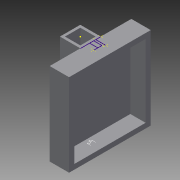
# Autodesk Inventor part: CouterWeightLink
Saved by Autodesk Inventor 2015 (Build 190159000, 159)
## iProperties
Created: 2016-03-24
Part Number: CouterWeightLink
Material: Generic
Document SubType Name: Modeling
Designer: Hatch
Density: 1 g/cm^3
Appearance: Default
Author: Hatch
Autodesk Inventor part; units mm, degrees
ref_plane "YZ Plane" through (0, 0, 0) normal (1, 0, 0) x (0, 1, 0)
ref_plane "XZ Plane" through (0, 0, 0) normal (0, 1, 0) x (-1, 0, 0)
ref_plane "XY Plane" through (0, 0, 0) normal (0, 0, 1) x (1, 0, 0)
sketch "Sketch1" plane through (0, 0, 0) normal (0, 1, 0) x (-1, 0, 0)
  line L0 (-7.25, 7.25) -> (7.25, 7.25)
  line L1 (7.25, 7.25) -> (7.25, -7.25)
  line L2 (7.25, -7.25) -> (-7.25, -7.25)
  line L3 (-7.25, -7.25) -> (-7.25, 7.25)
  line L4 (-7.25, 7.25) -> (7.25, -7.25) construction
  line L5 (7.25, 7.25) -> (-7.25, -7.25) construction
  point P0 (0, 0)
  dimension "d0" = 14.5
  dimension "d1" = 14.5
  constraints: 12 end point, 2 midpoint, 2 parallel, 1 horizontal, 1 perpendicular
  measures "d0" distance of L1.end L2.end
  measures "d1" distance of L0.end L1.end
extrude "Extrusion1" add sketch "Sketch1" along normal blind 76.2
sketch "Sketch2" plane through (0, 76.2, 0) normal (0, 1, 0) x (1, 0, 0)
  line L0 (10, -10) -> (-10, -10)
  line L1 (-10, -10) -> (-10, 10)
  line L2 (-10, 10) -> (10, 10)
  line L3 (10, 10) -> (10, -10)
  line L4 (10, -10) -> (-10, 10) construction
  line L5 (-10, -10) -> (10, 10) construction
  point P0 (0, 0)
  dimension "d4" = 20
  dimension "d5" = 20
  constraints: 12 end point, 2 midpoint, 2 parallel, 1 horizontal, 1 perpendicular
  measures "d4" distance of L1.end L2.end
  measures "d5" distance of L0.end L1.end
extrude "Extrusion2" add sketch "Sketch2" along normal blind 5
sketch "Sketch3" plane through (0, 81.2, 0) normal (0, 1, 0) x (1, 0, 0)
  line L0 (7.5, -7.5) -> (-7.5, -7.5)
  line L1 (-7.5, -7.5) -> (-7.5, 7.5)
  line L2 (-7.5, 7.5) -> (7.5, 7.5)
  line L3 (7.5, 7.5) -> (7.5, -7.5)
  line L4 (7.5, -7.5) -> (-7.5, 7.5) construction
  line L5 (-7.5, -7.5) -> (7.5, 7.5) construction
  line L6 (10, -10) -> (-10, -10)
  line L7 (-10, -10) -> (-10, 10)
  line L8 (-10, 10) -> (10, 10)
  line L9 (10, 10) -> (10, -10)
  line L10 (10, -10) -> (-10, 10) construction
  line L11 (-10, -10) -> (10, 10) construction
  point P0 (0, 0)
  dimension "d8" = 15
  dimension "d9" = 15
  constraints: 24 end point, 4 midpoint, 4 parallel, 2 horizontal, 2 perpendicular
  measures "d8" distance of L1.end L2.end
  measures "d9" distance of L0.end L1.end
extrude "Extrusion3" add sketch "Sketch3" along normal blind 76.2
sketch "Sketch4" plane through (10, 76.2, 10) normal (1, 0, 0) x (0, 0, -1)
  line L0 (20, 0) -> (20, 81.2) projected
  line L1 (15, 81.2) -> (15, 0)
  line L2 (0, 0) -> (20, 0) projected
  line L3 (15, 81.2) -> (13, 81.2)
  line L4 (17.5, 81.2) -> (2.5, 81.2) projected
  line L5 (13, 81.2) -> (13, 0)
  line L6 (13, 0) -> (15, 0)
  line L7 (20, 81.2) -> (0, 81.2) projected
  point P0 (10, -76.2)
  dimension "d12" = 2
  constraints: 8 end point, 3 point on line, 1 parallel, 1 perpendicular, 1 vertical
  measures "d12" distance of L1.start L3.end
extrude "Extrusion4" add sketch "Sketch4" along normal blind 10 contours L2 L5 L3 L1
sketch "Sketch5" plane through (10, 76.2, -3) normal (0, 0, 1) x (1, 0, 0)
  line L0 (0, 81.2) -> (10, 81.2) projected
  line L1 (10, 81.2) -> (8, 81.2)
  line L2 (8, 81.2) -> (8, 0)
  line L3 (8, 0) -> (10, 0)
  line L4 (10, 0) -> (10, 81.2)
  point P0 (-10, -76.2)
  dimension "d15" = 2
  constraints: 8 end point, 2 parallel, 1 perpendicular, 1 point on line
  measures "d15" distance of L0.end L1.end
extrude "Extrusion5" add sketch "Sketch5" along normal blind 8
sketch "Sketch6" plane through (20, 76.2, 10) normal (1, 0, 0) x (0, 0, -1)
  line L0 (5, 81.2) -> (3, 81.2)
  line L1 (3, 81.2) -> (3, 0)
  line L2 (3, 0) -> (5, 0)
  line L3 (5, 0) -> (5, 81.2)
  point P0 (10, -76.2)
  dimension "d18" = 2
  constraints: 8 end point, 2 parallel, 1 horizontal, 1 perpendicular
  measures "d18" distance of L0.start L0.end
extrude "Extrusion6" add sketch "Sketch6" against normal blind 4
sketch "Sketch7" plane through (0, 157.4, 0) normal (0, 1, 0) x (1, 0, 0)
  line L0 (18, 3) -> (18, -5)
  line L1 (18, 3) -> (18, -5) projected
  line L2 (18, -1) -> (10, -1)
  line L3 (10, 3) -> (10, -10) projected
  line L4 (10, -10) -> (10, -1)
  line L5 (10, 10) -> (10, -1)
  line L6 (10, 5) -> (20, 5)
  line L7 (10, 3) -> (18, 3)
  line L8 (10, 3) -> (18, 3) projected
  point P0 (0, 0)
  constraints: 12 end point, 4 collinear, 2 horizontal, 1 midpoint, 1 point on line
sketch "Sketch8" plane through (0, 76.2, 0) normal (0, -1, 0) x (1, 0, 0)
  line L0 (16, 7) -> (16, 5)
  line L1 (16, 7) -> (16, 5) projected
  line L2 (18, 5) -> (18, -3)
  line L3 (18, -3) -> (18, 5) projected
  line L4 (16, 6) -> (16, 1)
  point P0 (0, 0)
  dimension "d21" = 5
  constraints: 6 end point, 2 collinear, 1 midpoint, 1 point on line
  measures "d21" distance of L4.start L4.end
sketch "Sketch9" plane through (7.25, 0, 7.25) normal (1, 0, 0) x (0, 0, -1)
  line L0 (0, 0) -> (14.5, 0)
  line L1 (14.5, 0) -> (14.5, 76.2)
  line L2 (14.5, 76.2) -> (0, 76.2)
  line L3 (0, 76.2) -> (0, 0)
  point P0 (7.25, 0)
  constraints: 8 end point, 2 parallel, 1 horizontal, 1 perpendicular
extrude "Extrusion7" cut sketch "Sketch9" against normal through all
sketch "Sketch10" plane through (0, 76.2, 0) normal (0, -1, 0) x (1, 0, 0)
  line L0 (10, -5) -> (20, -5)
  line L1 (20, -5) -> (20, 7)
  line L2 (20, 7) -> (10, 7)
  line L3 (10, 7) -> (10, -5)
  point P0 (0, 0)
  constraints: 8 end point, 2 parallel, 1 horizontal, 1 perpendicular
extrude "Extrusion8" cut sketch "Sketch10" against normal through all
sketch "Sketch11" plane through (10, 76.2, 10) normal (1, 0, 0) x (0, 0, -1)
  line L0 (20, 81.2) -> (50, 81.2)
  line L1 (0, 81.2) -> (-30, 81.2)
  line L2 (-30, 81.2) -> (50, 81.2)
  line L3 (50, 81.2) -> (50, 0.1684)
  line L4 (50, 0.1684) -> (-30, 0.1684)
  line L5 (-30, 0.1684) -> (-30, 81.2)
  point P0 (10, -76.2)
  dimension "d26" = 30
  dimension "d27" = 30
  constraints: 12 end point, 3 horizontal, 2 parallel, 1 perpendicular
  measures "d26" distance of L0.start L0.end
  measures "d27" distance of L1.start L1.end
extrude "Extrusion9" add sketch "Sketch11" along normal blind 4
sketch "Sketch12" plane through (14, 76.2, 10) normal (1, 0, 0) x (0, 0, -1)
  line L0 (0, 81.2) -> (0, 76.2)
  line L1 (0, 0) -> (0, 81.2) projected
  line L2 (0, 66.0511) -> (-25, 66.0511)
  line L3 (-30, 81.2) -> (-30, 0.1684) projected
  line L4 (0, 25.128) -> (45, 25.128)
  line L5 (50, 0.1684) -> (50, 81.2) projected
  line L6 (31.5529, 0) -> (31.5529, 5)
  line L7 (-25, 76.2) -> (45, 76.2)
  line L8 (45, 76.2) -> (45, 5)
  line L9 (45, 5) -> (-25, 5)
  line L10 (-25, 5) -> (-25, 76.2)
  line L11 (-30, 81.2) -> (50, 81.2)
  line L12 (50, 81.2) -> (50, 0.1684)
  line L13 (50, 0.1684) -> (-30, 0.1684)
  line L14 (-30, 0.1684) -> (-30, 81.2)
  point P0 (10, -76.2)
  dimension "d30" = 5
  dimension "d31" = 25
  dimension "d32" = 45
  dimension "d33" = 5
  constraints: 24 end point, 4 parallel, 4 perpendicular, 3 point on line, 2 horizontal, 1 vertical
  measures "d30" distance of L0.start L0.end
  measures "d31" distance of L2.start L2.end
  measures "d32" distance of L4.start L4.end
  measures "d33" distance of L6.start L6.end
extrude "Extrusion10" add sketch "Sketch12" along normal blind 15 contours L11 L5 L13 L6 L9 L8 L7 L0 | L0 L7 L10 L9 L1 L13 L3 L11 | L1 L9 L6 L13
body "Solid1"
